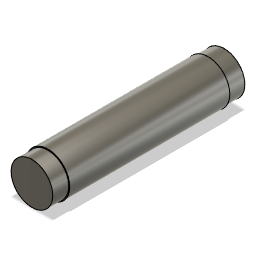
Torque+rod (Autodesk Fusion 360 design; units mm, degrees)
Autodesk Fusion 360 part; units mm, degrees
sketch "Sketch1" plane through (0, 0, 0) normal (0, 0, 1) x (1, 0, 0)
  circle A0 centre (0, 0) radius 6.5
  circle A1 centre (0, 0) radius 6.8
  dimension "d6" = 13
  dimension "d7" = 13.6
  constraint coincident A0.centre A1.centre
  measures "d6" diameter of A0
  measures "d7" diameter of A1
extrude "Extrude1" add sketch "Sketch1" along normal blind 30 and the other way blind 30 contours A0
extrude "Extrude2" add sketch "Sketch1" along normal mid plane 50
